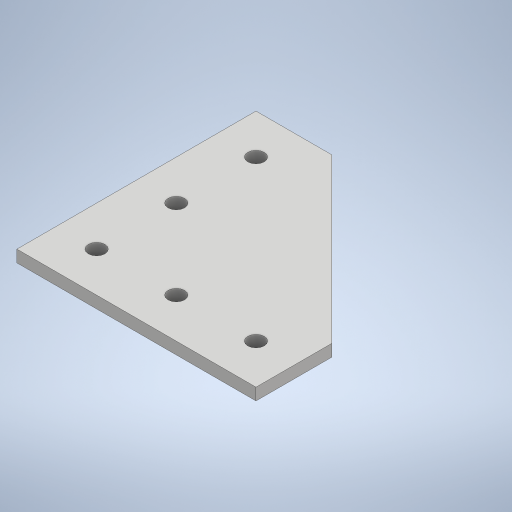
# Autodesk Inventor part: escuadra plana
Saved by Autodesk Inventor 2024.2 (Build 282272000, 272)
## iProperties
Created: 2025-07-02
Part Number: escuadra plana
Material: Genérico
Document SubType Name: Modeling
Designer: jd.castellanosq
Density: 1 g/cm^3
Appearance: Valor por defecto
Author: jd.castellanosq
Autodesk Inventor part; units mm, degrees
ref_plane "YZ Plane" through (0, 0, 0) normal (1, 0, 0) x (0, 1, 0)
ref_plane "XZ Plane" through (0, 0, 0) normal (0, 1, 0) x (-1, 0, 0)
ref_plane "XY Plane" through (0, 0, 0) normal (0, 0, 1) x (1, 0, 0)
sketch "Boceto1" plane through (0, 0, 0) normal (0, 0, 1) x (1, 0, 0)
  line L0 (0, 0) -> (0, 120)
  line L1 (0, 120) -> (38, 120)
  line L2 (38, 120) -> (120, 38)
  line L3 (120, 38) -> (120, 0)
  line L4 (120, 0) -> (0, 0)
  circle A0 centre (20, 20) radius 4.15
  circle A1 centre (20, 60) radius 4.15
  circle A2 centre (20, 100) radius 4.15
  circle A3 centre (60, 20) radius 4.15
  circle A4 centre (100, 20) radius 4.15
  dimension "d0" = 120
  dimension "d1" = 120
  dimension "d2" = 38
  dimension "d3" = 38
  dimension "d4" = 8.3
  dimension "d5" = 20
  dimension "d6" = 20
  dimension "d7" = 40
  dimension "d8" = 40
  dimension "d9" = 40
  dimension "d10" = 40
  constraints: 10 end point, 5 centre point, 4 equal radius, 2 horizontal alignment, 2 perpendicular, 2 vertical alignment, 1 parallel, 1 vertical
  measures "d0" distance of L0.start L0.end
  measures "d1" distance of L3.end L0.start
  measures "d2" distance of L0.end L1.end
  measures "d3" distance of L2.end L3.end
  measures "d4" diameter of A2
  measures "d5" distance from line of L0 A2.centre
  measures "d6" distance from line of A0.centre L4
  measures "d7" distance of A2.centre A1.centre
  measures "d8" distance of A1.centre A0.centre
  measures "d9" distance of A3.centre A0.centre
  measures "d10" distance of A4.centre A3.centre
extrude "Extrusión1" add sketch "Boceto1" along normal blind 6
equation "\"d9\" = d8"
equation "\"d10\" = d9"
